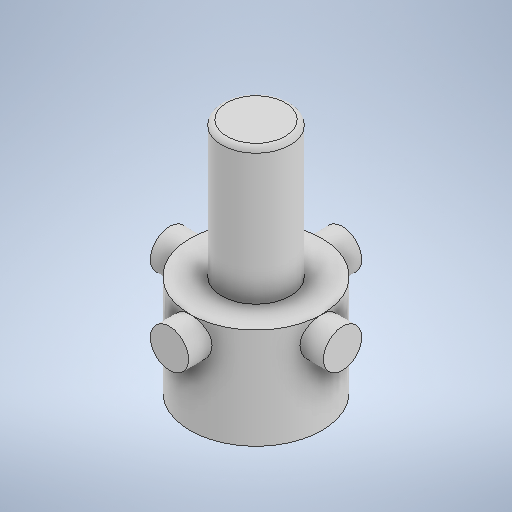
# Autodesk Inventor part: botao
Saved by Autodesk Inventor 2025.3 (Build 293356000, 356)
## iProperties
Created: 2025-07-28
Part Number: botao
Material: Genérico
Document SubType Name: Modeling
Designer: user
Density: 1 g/cm^3
Appearance: Padrão
Author: user
## iProperties of the stored document botao_3DPrint.ipt
Created: 2025-07-28
Part Number: botao_3DPrint
Material: Genérico
Document SubType Name: Modeling
Designer: user
Density: 1 g/cm^3
Appearance: Padrão
Author: user
Autodesk Inventor part; units mm, degrees
ref_plane "YZ Plane" through (0, 0, 0) normal (1, 0, 0) x (0, 1, 0)
ref_plane "XZ Plane" through (0, 0, 0) normal (0, 1, 0) x (-1, 0, 0)
ref_plane "XY Plane" through (0, 0, 0) normal (0, 0, 1) x (1, 0, 0)
sketch "Esboço1" plane through (0, 0, 0) normal (0, 0, 1) x (1, 0, 0)
  line L0 (0, 0) -> (6.55, 0)
  line L1 (6.55, 0) -> (6.55, 10)
  line L2 (6.55, 10) -> (3.4, 10)
  line L3 (3.4, 10) -> (3.4, 23.5)
  line L4 (3.4, 23.5) -> (0, 23.5)
  line L5 (0, 23.5) -> (0, 0)
  dimension "d0" = 6.55
  dimension "d1" = 10
  dimension "d3" = 13.5
  dimension "d14" = 3.4
  constraints: 12 end point, 4 perpendicular, 2 horizontal, 1 vertical
  measures "d0" distance of L0.start L0.end
  measures "d1" distance of L0.end L1.end
  measures "d3" distance of L2.end L3.end
  measures "d14" distance between parallel lines of L5 L3
revolve "Revolução1" add sketch "Esboço1" angle 360 about axis through (0, 23.5, 0) along (0, -1, 0)
sketch "Esboço2" plane through (0, 0, 0) normal (0, 0, 1) x (1, 0, 0)
  line L0 (-6.55, 10) -> (6.55, 10) projected
  line L1 (0, 10) -> (0, 8.1)
  circle A0 centre (0, 8.1) radius 1.9
  point P0 (0, 0)
  dimension "d11" = 3.8
  dimension "d5" = 1.9
  constraints: 2 end point, 1 coincident, 1 midpoint, 1 vertical, 1 vertical alignment, 2 other
  measures "d5" distance of L1.start L1.end
extrude "Extrusão1" add sketch "Esboço2" along normal mid plane 17.2
sketch "Esboço3" plane through (0, 0, 0) normal (1, 0, 0) x (0, 1, 0)
  line L0 (10, 3.4) -> (10, -3.4) projected
  line L1 (10, 0) -> (8.1, 0)
  circle A0 centre (8.1, 0) radius 1.9
  point P0 (0, 0)
  dimension "d8" = 1.9
  constraints: 2 end point, 1 coincident, 1 horizontal, 1 horizontal alignment, 1 midpoint, 2 other
  measures "d8" distance of L1.start L1.end
extrude "Extrusão2" add sketch "Esboço3" along normal mid plane 17.2
fillet "Arredondamento2" radius 0.5 1 edges at (-3.4, 23.5, 0)
